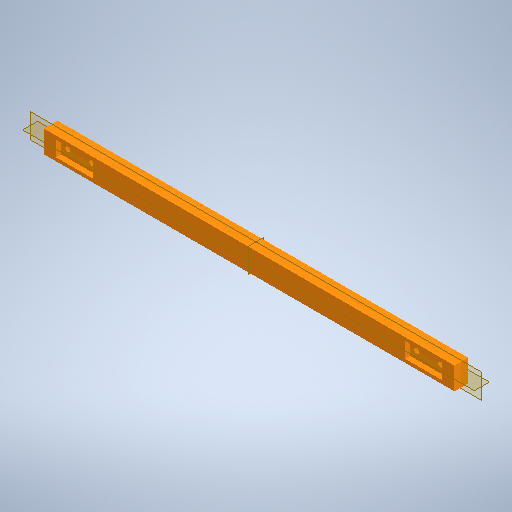
# Autodesk Inventor part: conector_eixos_001
Saved by Autodesk Inventor 2026 (Build 300175000, 175)
## iProperties
Created: 2025-11-27
Part Number: conector_eixos_001
Material: ABS Plastic
Document SubType Name: Modeling
Designer: Carlos Dias
Density: 1.06 g/cm^3
Appearance: Orange
Author: Carlos Dias
Autodesk Inventor part; units mm, degrees
sketch "Sketch1" plane through (0, 0, 0) normal (0, 0, 1) x (1, 0, 0)
  line L0 (-120, 6.5) -> (120, 6.5)
  line L1 (120, 6.5) -> (120, -6.5)
  line L2 (120, -6.5) -> (-120, -6.5)
  line L3 (-120, -6.5) -> (-120, 6.5)
  line L4 (-120, 6.5) -> (120, -6.5) construction
  line L5 (120, 6.5) -> (-120, -6.5) construction
  point P0 (0, 0)
  point P1 (0, 0)
  dimension "d0" = 240
  dimension "d1" = 13
  constraints: 12 end point, 2 midpoint, 2 parallel, 1 coincident, 1 horizontal, 1 perpendicular
  measures "d0" distance of L0.start L0.end
  measures "d1" distance of L0.end L1.end
extrude "Extrusion1" add sketch "Sketch1" along normal mid plane 8
sketch "Sketch2" plane through (0, 0, 4) normal (0, 0, 1) x (1, 0, 0)
  circle A0 centre (-109, 0) radius 1.5 projected
  circle A1 centre (-95, 0) radius 1.5 projected
  circle A2 centre (95, 0) radius 1.5 projected
  circle A3 centre (109, 0) radius 1.5 projected
  point P0 (0, 0)
extrude "Extrusion2" cut sketch "Sketch2" against normal through all
sketch "Sketch3" plane through (0, 0, 4) normal (0, 0, 1) x (1, 0, 0)
  line L0 (-95, 0) -> (-109, 0) construction
  circle A0 centre (-95, 0) radius 1.5 projected
  circle A1 centre (-109, 0) radius 1.5 projected
  line L1 (-91, 4.5) -> (-113, 4.5)
  line L2 (-113, 4.5) -> (-113, -4.5)
  line L3 (-113, -4.5) -> (-91, -4.5)
  line L4 (-91, -4.5) -> (-91, 4.5)
  line L5 (-91, 4.5) -> (-113, -4.5) construction
  line L6 (-113, 4.5) -> (-91, -4.5) construction
  circle A2 centre (109, 0) radius 1.5 projected
  circle A3 centre (95, 0) radius 1.5 projected
  line L7 (109, 0) -> (95, 0) construction
  line L8 (113, 4.5) -> (91, 4.5)
  line L9 (91, 4.5) -> (91, -4.5)
  line L10 (91, -4.5) -> (113, -4.5)
  line L11 (113, -4.5) -> (113, 4.5)
  line L12 (113, 4.5) -> (91, -4.5) construction
  line L13 (91, 4.5) -> (113, -4.5) construction
  point P0 (0, 0)
  point P1 (-102, 0)
  point P2 (-102, 0)
  point P3 (102, 0)
  point P4 (102, 0)
  dimension "d9" = 22
  dimension "d10" = 9
  constraints: 28 end point, 6 coincident, 6 midpoint, 4 horizontal, 4 parallel, 2 equal length, 2 horizontal alignment, 2 perpendicular
  measures "d9" distance of L2.end L3.end
  measures "d10" distance of L3.end L1.start
extrude "Extrusion3" cut sketch "Sketch3" against normal blind 3
body "Solid1"
